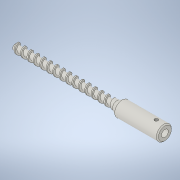
# Autodesk Inventor part: MC18_Welle
Saved by Autodesk Inventor 2021 (Build 250183000, 183)
## iProperties
Created: 2020-04-27
Part Number: MC18_Welle
Material: 1.4305
Document SubType Name: Modeling
Designer: kaebi
Density: 8 g/cm^3
Appearance: Stahl
Description: Dosierschnecke
Stock Number: BEF 012 A
Mass: 65.4465 g
Surface Area: 52.9702 cm^2
Volume: 8.18081 cm^3
Author: kaebi
Autodesk Inventor part; units mm, degrees
ref_plane "YZ Plane" through (0, 0, 0) normal (1, 0, 0) x (0, 1, 0)
ref_plane "XZ Plane" through (0, 0, 0) normal (0, 1, 0) x (-1, 0, 0)
ref_plane "XY Plane" through (0, 0, 0) normal (0, 0, 1) x (1, 0, 0)
sketch "Skizze1" plane through (0, 0, 0) normal (0, 0, 1) x (1, 0, 0)
  line L0 (-140, 0) -> (-26.9228, 0)
  line L1 (-26.9228, 0) -> (-25, 3.2)
  line L2 (-25, 3.2) -> (0, 3.2)
  line L3 (0, 3.2) -> (0, 7)
  line L4 (0, 7) -> (-40, 7)
  line L5 (-40, 7) -> (-45, 4)
  line L6 (-45, 4) -> (-140, 4)
  line L7 (-140, 4) -> (-140, 0)
  line L8 (-57.7817, 0) -> (41.8277, 0)
  point P0 (0, 0)
  dimension "d1" = 25
  dimension "d2" = 59
  dimension "d3" = 6.4
  dimension "d4" = 14
  dimension "d5" = 40
  dimension "d6" = 5
  dimension "d8" = 140
  dimension "d9" = 8
  constraints: 18 end point, 3 perpendicular, 2 horizontal, 2 parallel, 1 collinear, 1 point on line, 1 vertical alignment
  measures "d1" distance of L1.end L2.end
  measures "d2" angle of L8 L1
  measures "d3" diameter of L2 L8
  measures "d4" diameter of L4 L8
  measures "d5" distance of L3.end L4.end
  measures "d6" horizontal distance of L4.end L5.end
  measures "d8" distance between parallel lines of L7 L3
  measures "d9" diameter of L6 L8
revolve "Umdrehung1" add sketch "Skizze1" angle 360 about axis through (-57.7817, 0, 0) along (1, 0, 0)
sketch "Skizze2" plane through (0, 0, 0) normal (0, 1, 0) x (-1, 0, 0)
  line L0 (0, 7) -> (0, -7) projected
  point P0 (0, 0)
  point P1 (8, 0)
  point P2 (0, 0)
  dimension "d10" = 8
  constraints: 1 horizontal alignment, 1 midpoint
  measures "d10" distance from line of L0 point (8, 0)
hole "Bohrung1" at (-8, 0, 0) direction (0, 1, 0) diameter 3.242 end through all thread size "M4x0.7" class "6H" standard "ISO Metric profile"
chamfer "Fase1" distance 1 angle 45 1 edges at (0, -7, 0)
sketch "Skizze3" plane through (0, 0, 0) normal (0, 1, 0) x (-1, 0, 0)
  line L0 (140, 4) -> (140, -4) projected
  line L1 (140, 0) -> (144.6075, 0)
  line L2 (140, -4) -> (45, -4) projected
  line L3 (140, -4) -> (145, -4)
  line L4 (145, -4) -> (144.8025, -2.5)
  line L5 (144.8025, -2.5) -> (140.1975, -2.5)
  line L6 (140.1975, -2.5) -> (140, -4)
  point P0 (0, 0)
  dimension "d32" = 5
  dimension "d33" = 5
  dimension "d35" = 15
  constraints: 10 end point, 2 horizontal, 1 equal length, 1 midpoint
  measures "d32" diameter of L5 L1
  measures "d33" distance of L2.start L3.end
  measures "d35" angle of L4 L6
coil "Spirale1" sketch "Skizze3" operation cut axis through (-140, 0, 0) along (1, 0, 0) pitch 6 turns 15.833333 hand right
